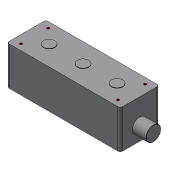
# Autodesk Inventor part: TL20240701-3구 스위치 박스
Saved by Autodesk Inventor 2022.5 (Build 265521000, 521)
## iProperties
Category: SUB ASSEMBLY NAME
Company: 고객사
Created: 2023-09-09
Part Number: TL20240701-3구 스위치 박스
Checked By: 작성자
Engr Approved By: 윤수현
User Status: 수량ea / set
Material: 일반
Document SubType Name: Modeling
Mfg Approved By: 호상태
Designer: 길창현
Stock Number: 부품 번호
Density: 1 g/cm^3
Appearance: 기본값
DETAIL: Coveryor Assembly
M/C TITLE: CJ 제일제당 협동로봇 포장시스탬 PILOT 장비
PARTS NAME: Bracket
SPECIFICATION: TA20221101-CV200000-015
DocNumber: 221118_Standard_v1
Folder: .\
VDS_Category: 엔지니어링
Title: 도면 명
Subject: 프로젝트 명
Author: 길창현
Revision Number: A
Autodesk Inventor part; units mm, degrees
ref_plane "YZ Plane" through (0, 0, 0) normal (1, 0, 0) x (0, 1, 0)
ref_plane "XZ Plane" through (0, 0, 0) normal (0, 1, 0) x (-1, 0, 0)
ref_plane "XY Plane" through (0, 0, 0) normal (0, 0, 1) x (1, 0, 0)
sketch "스케치9" plane through (0, 0, 0) normal (0, 0, 1) x (1, 0, 0)
  line L0 (-125, 43) -> (125, 43)
  line L1 (125, 43) -> (125, -43)
  line L2 (125, -43) -> (-125, -43)
  line L3 (-125, -43) -> (-125, 43)
  line L4 (-125, 43) -> (125, -43) construction
  line L5 (125, 43) -> (-125, -43) construction
  point P0 (0, 0)
  dimension "d40" = 250
  dimension "d41" = 86
  constraints: 12 end point, 2 midpoint, 2 parallel, 1 horizontal, 1 perpendicular
  measures "d40" distance of L0.start L0.end
  measures "d41" distance between parallel lines of L2 L0
extrude "돌출4" add sketch "스케치9" along normal blind 85
fillet "모깎기2" radius 5 4 edges at (125, -43, 42.5) (125, 43, 42.5) (-125, -43, 42.5) (-125, 43, 42.5)
sketch "스케치10" plane through (0, 0, 0) normal (0, 0, -1) x (-1, 0, 0)
  point P0 (0, 0)
  point P1 (107, 30)
  point P2 (-107, 30)
  point P3 (-107, -30)
  point P4 (107, -30)
  dimension "d45" = 214
  dimension "d46" = 60
  dimension "d47" = 107
  dimension "d48" = 30
  constraints: 2 horizontal alignment, 2 vertical alignment
  measures "d45" distance of point (-107, -30) point (107, -30)
  measures "d46" distance of point (107, 30) point (107, -30)
  measures "d47" horizontal distance of point (0, 0) point (107, -30)
  measures "d48" vertical distance of point (107, -30) point (0, 0)
hole "구멍3" at (-107, 30, 0) at (107, 30, 0) at (107, -30, 0) at (-107, -30, 0) direction (0, 0, 1) diameter 5.5 end through all clearance for "Socket Head Cap Screw" size "M5" standard "TS Profile"
sketch "스케치11" plane through (0, 0, 85) normal (0, 0, 1) x (1, 0, 0)
  circle A0 centre (0, 0) radius 12.5
  circle A1 centre (0, 0) radius 12.5
  circle A2 centre (-75, 0) radius 12.5
  circle A3 centre (75, 0) radius 12.5
  dimension "d56" = 0
  dimension "d57" = 25
  dimension "d58" = 0
  dimension "d61" = 25
  dimension "d62" = 25
  dimension "d63" = 75
  dimension "d64" = 75
  constraints: 4 centre point, 2 coincident, 2 horizontal alignment, 1 concentric
  measures "d56" distance of A1.centre A0.centre
  measures "d57" diameter of A0
  measures "d58" distance of point (0, 0) A0.centre
  measures "d61" diameter of A2
  measures "d62" diameter of A3
  measures "d63" distance of A0.centre A2.centre
  measures "d64" distance of A1.centre A3.centre
extrude "돌출5" add sketch "스케치11" along normal blind 1
sketch "Sketch12" plane through (125, -38, 0) normal (1, 0, 0) x (0, 0, -1)
  circle A0 centre (-30, 38) radius 16.25
  line L0 (0, 0) -> (0, 76) projected
  point P0 (0, 38)
  point P1 (0, 38)
  dimension "d65" = 32.5
  dimension "d66" = 30
  constraints: 1 centre point, 1 horizontal alignment, 1 midpoint
  measures "d65" diameter of A0
  measures "d66" distance from line of A0.centre L0
extrude "Extrusion6" add sketch "Sketch12" along normal blind 30.5
chamfer "Chamfer1" distance 0.5 angle 45 1 edges at (155.5, 0, 46.25)
equation "\"d47\" = 0.5 * d45"
equation "\"d48\" = 0.5 * d46"
equation "\"d63\" = d64"
